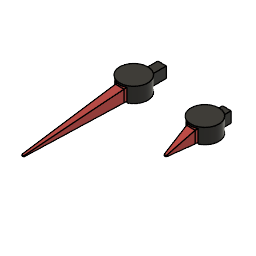
Zeiger (Autodesk Fusion 360 design; units mm, degrees)
Autodesk Fusion 360 part; units mm, degrees
note: some values were not read from the file. Set by a fixed rule: which sketch regions a step uses.
sketch "Sketch1" plane through (0, 0, 0) normal (0, 1, 0) x (1, 0, 0)
  circle A0 centre (0, 0) radius 6.5
  line L0 (0, 0) -> (2, 0)
  line L1 (2, 0) -> (-2, 0)
  line L2 (-2, 0) -> (-2, 6.1847)
  line L3 (2, 0) -> (2, 6.1847)
  line L4 (2, 6.1847) -> (2, 13.1847)
  line L5 (-2, 6.1847) -> (-2, 13.1847)
  line L6 (-2, 13.1847) -> (2, 13.1847)
  line L7 (0, -6.5) -> (0, -51.5)
  line L8 (0, -51.5) -> (-0.5, -51.5)
  line L9 (0, -51.5) -> (0.5, -51.5)
  line L10 (0, -6.5) -> (2, -6.5)
  line L11 (0, -6.5) -> (-2, -6.5)
  line L12 (2, -6.5) -> (0.5, -51.5)
  line L13 (-0.5, -51.5) -> (-2, -6.5)
  line L14 (2, -6.5) -> (2, -2.8723)
  line L15 (-2, -6.5) -> (-2, -2.8723)
  circle A1 centre (0, 0) radius 3.5
  circle A2 centre (0, 0) radius 4.25
  line L16 (2.75, -6.5) -> (2.75, -2.8723)
  line L17 (-2.75, -6.5) -> (-2.75, -2.8723)
  circle A3 centre (33, 0) radius 6.5
  line L18 (35, 0) -> (31, 0)
  line L19 (35, 0) -> (35, 6.1847)
  line L20 (31, 10.1847) -> (35, 10.1847)
  line L21 (31, 6.1847) -> (31, 10.1847)
  line L22 (31, 0) -> (31, 6.1847)
  line L23 (35, 6.1847) -> (35, 10.1847)
  circle A4 centre (33, 0) radius 4.25
  circle A5 centre (33, 0) radius 3.5
  line L24 (35.75, -6.5) -> (35.75, -2.8723)
  line L25 (30.25, -6.5) -> (30.25, -2.8723)
  line L26 (31, -6.5) -> (31, -2.8723)
  line L27 (35, -6.5) -> (35, -2.8723)
  line L28 (33, 0) -> (33, -6.5)
  line L29 (33, -6.5) -> (33, -18.5)
  line L30 (33, -18.5) -> (32.5, -18.5)
  line L31 (33, -18.5) -> (33.5, -18.5)
  line L32 (33.5, -18.5) -> (35, -6.5)
  line L33 (32.5, -18.5) -> (31, -6.5)
  dimension "d1" = 13
  dimension "d2" = 2
  dimension "d3" = 4
  dimension "d4" = 7
  dimension "d9" = 45
  dimension "d10" = 0.5
  dimension "d11" = 0.5
  dimension "d12" = 2
  dimension "d13" = 2
  dimension "d14" = 7
  dimension "d15" = 0.75
  dimension "d16" = 0.75
  dimension "d17" = -0.75
  dimension "d25" = 0.75
  dimension "d26" = 0.75
  dimension "d27" = -0.75
  dimension "d28" = 13
  dimension "d29" = 4
  dimension "d30" = 4
  dimension "d33" = 7
  dimension "d34" = 12
  dimension "d35" = 0.5
  dimension "d36" = 0.5
  constraint coincident A0.centre L0.start
  constraint horizontal L0
  constraint parallel L0 L1
  constraint coincident A0 L2.end
  constraint perpendicular L1 L2
  constraint coincident A0 L3.end
  constraint perpendicular L1 L3
  constraint perpendicular L1 L4
  constraint parallel L2 L5
  constraint perpendicular L2 L6
  constraint coincident A0 L7.start
  constraint vertical L7
  constraint perpendicular L7 L8
  constraint perpendicular L7 L9
  constraint tangent A0 L10
  constraint perpendicular L7 L10
  constraint tangent A0 L11
  constraint perpendicular L10 L14
  constraint perpendicular L11 L15
  constraint coincident L14.end A1
  constraint coincident L15.end A1
  constraint coincident L21.start A3
  constraint perpendicular L18 L22
  constraint coincident L19.end A3
  constraint perpendicular L18 L19
  constraint perpendicular L18 L23
  constraint parallel L21 L22
  constraint perpendicular L20 L22
  constraint coincident L27.end A5
  constraint coincident L26.end A5
  constraint coincident A3.centre A4.centre
  constraint coincident A3 L28.end
  constraint vertical L28
  constraint parallel L28 L29
  constraint perpendicular L28 L30
  constraint perpendicular L29 L31
  measures "d1" diameter of A0
  measures "d2" distance of A0.centre L0.end
  measures "d3" distance of L0.end L1.end
  measures "d4" distance of L3.end L4.end
  measures "d9" distance of L7.start L7.end
  measures "d10" distance of L7.end L8.end
  measures "d11" distance of L7.end L9.end
  measures "d12" distance of L7.start L10.end
  measures "d13" distance of L7.start L11.end
  measures "d14" diameter of A1
  measures "d28" diameter of A3
  measures "d29" distance of L18.end L18.start
  measures "d30" distance of L19.end L20.end
  measures "d33" diameter of A5
  measures "d34" distance of L28.end L29.end
  measures "d35" distance of L29.end L30.end
  measures "d36" distance of L29.end L31.end
extrude "Extrude1" add sketch "Sketch1" along normal blind 7 contours A0 L3 A2 L16 | A0 L2 L3 A2 | A0 L2 A2 L17 | A3 L19 A4 L24 | A3 L19 L22 A4 | A3 L22 A4 L25 makes body 1 at (3.8388, 4.6667, 5.2454) makes body 2 at (36.3101, 2.3333, 5.594)
extrude "Extrude2" add sketch "Sketch1" along normal blind 5 contours A0 L4 L5 L6 | A3 L20 L21 L23 bodies 1 2
extrude "Extrude3" add sketch "Sketch1" against normal blind 0.75 from surface at 7 contours A0 L14 A2 L16 | L3 L14 A1 A2 | L2 L3 A1 A2 | A0 L14 L15 A2 | A0 L15 A2 L17 | L2 L15 A1 A2 | L0 L1 L2 L3 A1 | L0 L1 L2 L3 A1 | L14 L15 A1 A2 | A3 A4 L24 L27 | L19 A4 A5 L27 | L19 L22 A4 A5 | A3 A4 L27 L28 | A3 A4 L25 L26 | L22 A4 A5 L26 | L18 L19 A5 L28 | L18 L19 L22 A5 | A3 A4 L26 L28 | A4 A5 L27 L28 | L18 L22 A5 L28 | A4 A5 L26 L28 bodies 1 2
extrude "Extrude4" add sketch "Sketch1" along normal blind 5.5 separate body contours A0 L10 L14 | A0 L14 L15 A2 | L0 L1 L2 L3 A1 | L0 L1 L2 L3 A1 | A0 L11 L15 | L7 L9 L10 L12 | L7 L8 L11 L13 | L14 L15 A1 A2 | A3 L27 L29 L31 L32 | A3 A4 L27 L28 | L18 L19 A5 L28 | L18 L19 L22 A5 | A3 L26 L29 L30 L33 | A3 A4 L26 L28 | A4 A5 L27 L28 | L18 L22 A5 L28 | A4 A5 L26 L28 makes body 3 at (1.5, 1.8333, 21.5) makes body 4 at (35.275, 3.6667, 2.6598)
chamfer "Chamfer1" distance 45 distance2 5 1 edges at (0, 5.5, 51.5) measured on face at (0.1667, 5.5, 21.5) on bodies 3
chamfer "Chamfer2" distance 12 distance2 5 1 edges at (33, 5.5, 18.5) measured on face at (32.8333, 5.5, 10.5) on bodies 4
named bodies: "BigMain", "BigZeiger", "SmallMain", "SmallZeiger"
